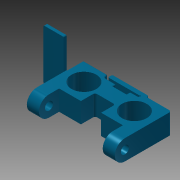
# Autodesk Inventor part: CounterWeightLoop2
Saved by Autodesk Inventor 2014 SP1 (Build 180222100, 222)
## iProperties
Created: 2016-11-30
Part Number: CounterWeightLoop2
Material: Generic
Document SubType Name: Modeling
Designer: danielsikar
Density: 1 g/cm^3
Appearance: Sky Blue Dark
Author: danielsikar
Autodesk Inventor part; units mm, degrees
ref_plane "YZ Plane" through (0, 0, 0) normal (1, 0, 0) x (0, 1, 0)
ref_plane "XZ Plane" through (0, 0, 0) normal (0, 1, 0) x (-1, 0, 0)
sketch "Sketch1" plane through (0, 0, 0) normal (0, 0, 1) x (1, 0, 0)
  line L0 (0, 0) -> (33, 0)
  line L1 (33, 18) -> (0, 18)
  line L2 (0, 18) -> (0, 0)
  circle A0 centre (9.3, 9) radius 6.15
  circle A1 centre (34.3, 9) radius 6.15
  line L3 (43.6, 18) -> (43.6, 0)
  line L4 (33, 0) -> (43.6, 0)
  line L5 (33, 18) -> (43.6, 18)
  dimension "d2" = 12.3
  dimension "d3" = 9.3
  dimension "d4" = 12.3
  dimension "d5" = 25
  constraints: 12 end point, 3 parallel, 2 centre point, 1 horizontal, 1 perpendicular
  measures "d2" diameter of A0
  measures "d3" distance from line of A0.centre L2
  measures "d4" diameter of A1
  measures "d5" distance of A1.centre A0.centre
extrude "Extrusion1" add sketch "Sketch1" along normal blind 10
sketch "Sketch2" plane through (0, 0, 10) normal (0, 0, 1) x (1, 0, 0)
  line L0 (0, 0) -> (43.6, 0) projected
  line L1 (43.6, 18) -> (0, 18) projected
  line L2 (21.8, 18) -> (21.8, 0) construction
  arc A0 (16.1431, 7) -> (18.3, 13.8734) centre (21.8, 9) ccw construction
  line L3 (18.3, 14.1204) -> (25.3, 14.1204)
  line L4 (18.3, 16.9204) -> (25.3, 16.9204)
  line L5 (25.3, 20.5535) -> (25.3, 9) construction
  line L6 (18.3, 20.5535) -> (18.3, 10.3573) construction
  line L7 (16.8, 0) -> (26.8, 0)
  line L8 (26.8, 0) -> (26.8, 7)
  line L9 (26.8, 7) -> (16.8, 7)
  line L10 (16.8, 7) -> (16.8, 0)
  line L11 (18.3, 13.8734) -> (18.3, 16.9204)
  line L12 (25.3, 16.9204) -> (25.3, 14.1204)
  line L13 (18.3, 16.9204) -> (25.3, 16.9204)
  line L14 (25.3, 16.9204) -> (25.3, 14.1204)
  line L15 (25.3, 14.1204) -> (18.3, 14.1204)
  line L16 (18.3, 14.1204) -> (18.3, 16.9204)
  line L17 (16.8, 7) -> (26.8, 7)
  line L18 (26.8, 7) -> (26.8, 0)
  line L19 (26.8, 0) -> (16.8, 0)
  line L20 (16.8, 0) -> (16.8, 7)
  dimension "d9" = 12
  dimension "d10" = 2.8
  dimension "d11" = 3.5
  dimension "d12" = 3.5
  dimension "d13" = 2
  dimension "d62" = 10
  dimension "d63" = 5
  constraints: 38 end point, 8 parallel, 7 point on line, 5 perpendicular, 3 horizontal, 3 midpoint, 2 point on circle, 1 centre point
  measures "d9" diameter of A0
  measures "d10" distance between parallel lines of L4 L3
  measures "d11" distance between parallel lines of L5 L2
  measures "d12" distance between parallel lines of L2 L6
  measures "d13" distance from line of L9 A0.centre
  measures "d62" distance between parallel lines of L8 L10
  measures "d63" distance between parallel lines of L2 L8
extrude "Extrusion2" cut sketch "Sketch2" against normal blind 10
fillet "Fillet1" radius 1 3 edges at (16.8, 7, 5) (26.8, 7, 5) (43.6, 18, 5)
sketch "Sketch3" plane through (0, 0, 10) normal (0, 0, 1) x (1, 0, 0)
  line L0 (18.3, 16.9204) -> (12.3, 16.9204)
  line L1 (12.3, 16.9204) -> (12.3, 15.9866)
  line L2 (12.3, 15.9866) -> (18.3, 15.9866)
  line L3 (18.3, 15.9866) -> (18.3, 16.9204)
  point P0 (0, 0)
  dimension "d17" = 6
  constraints: 8 end point, 2 parallel, 1 horizontal, 1 perpendicular
  measures "d17" distance between parallel lines of L1 L3
extrude "Extrusion3" cut sketch "Sketch3" against normal blind 10
sketch "Sketch4" plane through (0, 0, 10) normal (0, 0, 1) x (1, 0, 0)
  line L0 (42.6, 18) -> (0, 18) projected
  line L1 (12.3, 16.9204) -> (13.3, 16.9204)
  line L2 (13.3, 16.9204) -> (13.3, 18)
  line L3 (13.3, 18) -> (12.3, 18)
  line L4 (12.3, 18) -> (12.3, 16.9204)
  point P0 (3, 18)
  point P1 (0, 0)
  dimension "d20" = 1
  constraints: 8 end point, 2 parallel, 1 horizontal, 1 perpendicular, 1 point on line
  measures "d20" distance of L3.end L2.end
extrude "Extrusion4" cut sketch "Sketch4" against normal blind 10
sketch "Sketch5" plane through (42.6, 18, 10) normal (0, 1, 0) x (1, 0, 0)
  circle A0 centre (-26.3, 5) radius 1.15
  line L0 (-30.3, 0) -> (-30.3, 10) projected
  point P0 (-42.6, 10)
  dimension "d23" = 2.3
  dimension "d24" = 4
  constraints: 1 centre point
  measures "d23" diameter of A0
  measures "d24" distance from line of A0.centre L0
extrude "Extrusion5" cut sketch "Sketch5" against normal blind 6
fillet "Fillet3" radius 1 1 edges at (12.3, 15.9866, 5)
fillet "Fillet4" radius 1 1 edges at (12.3, 18, 5)
fillet "Fillet6" radius 0.5 1 edges at (18.3, 15.9866, 5)
ref_plane "Work Plane1" through (13.8, 18, 0.5) normal (0, 1, 0) x (1, 0, 0)
sketch "Sketch7" plane through (13.8, 18, 0.5) normal (0, 1, 0) x (1, 0, 0)
  circle A0 centre (2.5, -4.5) radius 1.15 projected
  line L0 (-0.4642, 0.5) -> (11.5358, 0.5)
  line L1 (11.5358, 0.5) -> (11.5358, -9.5)
  line L2 (11.5358, -9.5) -> (-0.4642, -9.5)
  line L3 (-0.4642, -9.5) -> (-0.4642, 0.5)
  point P0 (-13.8, 0.5)
  dimension "d38" = 12
  dimension "d39" = 10
  constraints: 8 end point, 2 parallel, 1 horizontal, 1 perpendicular
  measures "d38" distance of L1.end L2.end
  measures "d39" distance of L0.end L1.end
extrude "Extrusion7" add sketch "Sketch7" along normal blind 1
sketch "Sketch8" plane through (0, 0, 10) normal (0, 0, 1) x (1, 0, 0)
  line L0 (13.3, 16.9204) -> (25.3, 16.9204) projected
  line L1 (25.3, 16.9204) -> (25.3, 14.1204) projected
  line L2 (25.3, 16.9204) -> (29.3, 16.9204)
  line L3 (29.3, 16.9204) -> (29.3, 15.9204)
  line L4 (29.3, 15.9204) -> (25.3, 15.9204)
  line L5 (25.3, 15.9204) -> (25.3, 16.9204)
  point P0 (13.8, 16.9204)
  point P1 (24.8, 16.9204)
  point P2 (25.3, 16.4204)
  point P3 (0, 0)
  dimension "d42" = 4
  dimension "d43" = 1
  dimension "d44" = 0
  constraints: 9 end point, 2 parallel, 1 horizontal, 1 perpendicular
  measures "d42" distance of L3.end L4.end
  measures "d43" distance of L2.end L3.end
  measures "d44" distance between parallel lines of L0 L2
extrude "Extrusion8" cut sketch "Sketch8" against normal through all
sketch "Sketch9" plane through (0, 0, 10) normal (0, 0, 1) x (1, 0, 0)
  circle A0 centre (29.3, 16.9204) radius 0.25
  point P0 (0, 0)
  dimension "d47" = 0.5
  constraints: 1 centre point, 1 coincident
  measures "d47" diameter of A0
extrude "Extrusion9" cut sketch "Sketch9" against normal through all
sketch "Sketch10" plane through (25.3358, 18, 0) normal (1, 0, 0) x (0, 0, -1)
  line L0 (0, 0) -> (-10, 0) projected
  line L1 (0, 0) -> (0, 1) projected
  line L2 (-10, 1) -> (0, 1) projected
  line L3 (-10, 0) -> (-10, 1) projected
  point P0 (0, -18)
extrude "Extrusion10" add sketch "Sketch10" along normal blind 6
fillet "Fillet8" radius 0.5 1 edges at (25.3, 15.9204, 5)
fillet "Fillet9" radius 0.5 2 edges at (13.3358, 19, 5) (13.3, 16.9204, 5)
fillet "Fillet10" radius 0.5 2 edges at (31.3358, 19, 5) (31.3358, 18, 5)
fillet "Fillet11" radius 0.5 16 edges at (12.0071, 17.7071, 10) (12.3, 16.9933, 10) (12.5929, 16.2795, 10) (15.55, 15.9866, 10) (18.1536, 15.8402, 10) (18.3, 14.8035, 10) (13.3179, 18, 10) (5.65, 18, 10) (13.3179, 18, 0) (5.65, 18, 0) (12.0071, 17.7071, 0) (12.3, 16.9933, 0) (12.5929, 16.2795, 0) (15.55, 15.9866, 0) (18.1536, 15.8402, 0) (18.3, 14.8035, 0)
sketch "Sketch12" plane through (0, 1, 0) normal (-1, 0, 0) x (0, 0, 1)
  line L0 (0, 16.5) -> (0, -1) projected
  line L1 (10, 16.5) -> (10, -1) projected
  line L2 (0, 8.75) -> (10, 8.75)
  line L3 (10, 8.75) -> (10, 7.25)
  line L4 (10, 7.25) -> (0, 7.25)
  line L5 (0, 7.25) -> (0, 8.75)
  line L6 (0, -1) -> (10, -1) projected
  point P0 (0, 0)
  point P1 (10, -2.5)
  point P2 (1, -1)
  point P3 (9.5, -3)
  dimension "d56" = 1.5
  dimension "d59" = 9.75
  constraints: 8 end point, 2 parallel, 2 point on line, 1 horizontal, 1 perpendicular, 1 other
  measures "d56" distance of L2.end L3.end
extrude "Extrusion11" add sketch "Sketch12" along normal blind 10 contours L2 L1 L4 L0
sketch "Sketch13" plane through (0, 0, 10) normal (0, 0, 1) x (1, 0, 0)
  line L0 (-10, 9.75) -> (0, 9.75)
  line L1 (0, 9.75) -> (0, 8.25)
  line L2 (0, 8.25) -> (-10, 8.25)
  line L3 (-10, 8.25) -> (-10, 9.75)
  point P0 (0, 0)
  constraints: 8 end point, 2 parallel, 1 horizontal, 1 perpendicular
extrude "Extrusion12" add sketch "Sketch13" along normal blind 15
fillet "Fillet12" radius 0.5 5 edges at (0, 17.8536, 0.1464) (0, 18, 5) (0, 17.8536, 9.8536) (0, 13.625, 10) (0, 13.625, 0)
fillet "Fillet13" radius 0.5 3 edges at (-10, 9, 0) (-10, 9, 25) (0, 9, 25)
sketch "Sketch15" plane through (0.5, 0, 0) normal (0, -1, 0) x (1, 0, 0)
  line L0 (-0.5, 0) -> (16.3, 0) projected
  line L1 (-0.5, 10) -> (5.5, 10)
  line L2 (5.5, 10) -> (5.5, 0)
  line L3 (5.5, 0) -> (-0.5, 0)
  line L4 (-0.5, 0) -> (-0.5, 10)
  dimension "d71" = 6
  constraints: 8 end point, 2 parallel, 1 horizontal, 1 perpendicular, 1 point on line
  measures "d71" distance of L2.end L3.end
extrude "Extrusion14" add sketch "Sketch15" along normal blind 10
sketch "Sketch16" plane through (43.6, 0, 0) normal (0, -1, 0) x (1, 0, 0)
  line L0 (-16.8, 0) -> (0, 0) projected
  line L1 (0, 10) -> (-6, 10)
  line L2 (-6, 10) -> (-6, 0)
  line L3 (-6, 0) -> (0, 0)
  line L4 (0, 0) -> (0, 10)
  point P0 (-43.6, 0)
  dimension "d74" = 6
  constraints: 8 end point, 2 parallel, 1 horizontal, 1 perpendicular, 1 point on line
  measures "d74" distance of L3.end L2.end
extrude "Extrusion15" add sketch "Sketch16" along normal blind 10
sketch "Sketch17" plane through (43.6, 17, 10) normal (1, 0, 0) x (0, 0, -1)
  line L0 (10, -27) -> (0, -27) projected
  circle A0 centre (5, -22) radius 2
  point P0 (10, -17)
  dimension "d77" = 4
  dimension "d78" = 5
  constraints: 1 centre point
  measures "d77" diameter of A0
  measures "d78" distance from line of L0 A0.centre
extrude "Extrusion16" cut sketch "Sketch17" against normal through all
fillet "Fillet14" radius 5 4 edges at (40.6, -10, 10) (40.6, -10, 0) (3, -10, 10) (3, -10, 0)
body "Solid1"
